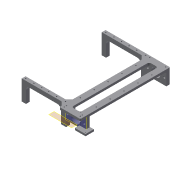
# Autodesk Inventor part: 02_Opentrons_Microscope_Base_v0
Saved by Autodesk Inventor 2019.4 (Build 234330000, 330)
## iProperties
Created: 2020-10-28
Part Number: 02_Opentrons_Microscope_Base_v0
Material: Generic
Document SubType Name: Modeling
Designer: diederichbenedict
Density: 1 g/cm^3
Appearance: Default
Author: diederichbenedict
Autodesk Inventor part; units mm, degrees
ref_plane "YZ Plane" through (0, 0, 0) normal (1, 0, 0) x (0, 1, 0)
ref_plane "XZ Plane" through (0, 0, 0) normal (0, 1, 0) x (-1, 0, 0)
ref_plane "XY Plane" through (0, 0, 0) normal (0, 0, 1) x (1, 0, 0)
ref_plane "Work Plane1" through (130.593, 54.6266, 280.0982) normal (0, 1, 0) x (1, 0, 0)
sketch "Sketch1" plane through (130.593, 54.6266, 280.0982) normal (0, 1, 0) x (1, 0, 0)
  line L0 (0, 36) -> (2, 38) projected
  line L1 (0, 27) -> (0, 36) projected
  line L2 (2, 25) -> (0, 27) projected
  line L3 (2, 25) -> (53, 25) projected
  line L4 (55, 27) -> (53, 25) projected
  line L5 (55, 27) -> (55, 36) projected
  line L6 (53, 38) -> (55, 36) projected
  line L7 (2, 38) -> (53, 38) projected
  circle A0 centre (6.5, 31.5) radius 2.5 construction
  circle A1 centre (48.5, 31.5) radius 2.5 construction
  line L8 (0, 224) -> (2, 226) projected
  line L9 (0, 215) -> (0, 224) projected
  line L10 (2, 213) -> (0, 215) projected
  line L11 (2, 213) -> (53, 213) projected
  line L12 (55, 215) -> (53, 213) projected
  line L13 (55, 215) -> (55, 224) projected
  line L14 (53, 226) -> (55, 224) projected
  line L15 (2, 226) -> (53, 226) projected
  circle A2 centre (6.5, 219.5) radius 2.5 construction
  circle A3 centre (48.5, 219.5) radius 2.5 construction
  line L16 (55, 25) -> (0, 25)
  line L17 (0, 25) -> (0, 261)
  line L18 (0, 261) -> (55, 261)
  line L19 (55, 261) -> (55, 25)
  line L20 (16, 261) -> (39, 261) projected
  circle A4 centre (48.5, 31.5) radius 1.45
  circle A5 centre (6.5, 31.5) radius 1.45
  circle A6 centre (48.5, 219.5) radius 1.45
  circle A7 centre (6.5, 219.5) radius 1.45
  point P0 (-130.593, 280.0982)
  dimension "d12" = 2.9
  dimension "d13" = 2.9
  dimension "d14" = 2.9
  dimension "d15" = 2.9
  constraints: 8 end point, 4 centre point, 3 coincident, 2 parallel, 2 point on line, 1 horizontal, 1 perpendicular
  measures "d12" diameter of A4
  measures "d13" diameter of A5
  measures "d14" diameter of A6
  measures "d15" diameter of A7
extrude "Extrusion1" add sketch "Sketch1" along normal blind 6
sketch "Sketch2" plane through (185.593, 54.6266, 19.0982) normal (0, 0, -1) x (-1, 0, 0)
  line L0 (46, 0) -> (46, 10) projected
  circle A0 centre (39, -26) radius 0.8 projected
  circle A1 centre (39, -3) radius 0.8 projected
  circle A2 centre (16, -26) radius 0.8 projected
  circle A3 centre (16, -3) radius 0.8 projected
  circle A4 centre (27.5, -14.5) radius 9.4 projected
  circle A5 centre (27.5, -14.5) radius 10.8 projected
  circle A6 centre (27.5, -14.5) radius 11.8
  circle A7 centre (5.5, -14.5) radius 3 projected
  circle A8 centre (49.5, -14.5) radius 3 projected
  circle A9 centre (5.5, -14.5) radius 3.1
  circle A10 centre (49.5, -14.5) radius 3.1
  line L1 (0, 0) -> (55, 0) projected
  line L2 (0, 0) -> (55, 0)
  line L3 (55, 0) -> (55, -32.5)
  line L4 (55, -32.5) -> (0, -32.5)
  line L5 (0, -32.5) -> (0, 0)
  point P0 (185.593, -54.6266)
  dimension "d2" = 1
  dimension "d3" = 6.2
  dimension "d4" = 6.2
  dimension "d5" = 18
  constraints: 8 end point, 3 centre point, 2 coincident, 2 parallel, 1 horizontal, 1 perpendicular
  measures "d2" radial gap between concentric circles of A5 A6
  measures "d3" diameter of A9
  measures "d4" diameter of A10
  measures "d5" distance from line of L4 A5.centre
extrude "Extrusion2" add sketch "Sketch2" against normal blind 10 contours L1 L3 L4 L5
ref_plane "Work Plane2" through (158.093, 40.1266, 239.5982) normal (0, 0, -1) x (1, 0, 0)
sketch "Sketch3" plane through (158.093, 40.1266, 239.5982) normal (0, 0, -1) x (1, 0, 0)
  circle A0 centre (-22, 0) radius 3 projected
  circle A1 centre (22, 0) radius 3 projected
  circle A2 centre (0, 0) radius 11.8 projected
  line L0 (27.5, -14.5) -> (27.5, -20.5) projected
  line L1 (-27.5, 18) -> (-27.5, -20.5) projected
  line L2 (27.5, -14.5) -> (-27.5, -14.5)
  line L3 (-27.5, -14.5) -> (-27.5, 15.5)
  line L4 (-27.5, 15.5) -> (27.5, 15.5)
  line L5 (27.5, 15.5) -> (27.5, -14.5)
  point P0 (-158.093, 40.1266)
  dimension "d51" = 30
  constraints: 8 end point, 2 parallel, 1 horizontal, 1 perpendicular, 1 point on line
  measures "d51" distance between parallel lines of L2 L4
extrude "Extrusion3" add sketch "Sketch3" along normal blind 10
fillet "Fillet1" radius 2 9 edges at (185.593, 41.3766, 19.0982) (158.093, 54.6266, 29.0982) (185.593, 39.6266, 229.5982) (185.593, 39.6266, 239.5982) (130.593, 39.6266, 229.5982) (130.593, 39.6266, 239.5982) (130.593, 57.6266, 255.0982) (185.593, 57.6266, 255.0982) (130.593, 41.3766, 19.0982)
sketch "Sketch4" plane through (130.593, 60.6266, 280.0982) normal (0, 1, 0) x (1, 0, 0)
  arc A0 (2, 261) -> (0, 259) centre (2, 259) ccw construction
  line L0 (0, 259) -> (0, 27) construction
  arc A1 (0, 27) -> (2, 25) centre (2, 27) ccw construction
  line L1 (2, 25) -> (53, 25) construction
  arc A2 (53, 25) -> (55, 27) centre (53, 27) ccw construction
  line L2 (55, 27) -> (55, 259) construction
  arc A3 (55, 259) -> (53, 261) centre (53, 259) ccw construction
  line L3 (53, 261) -> (2, 261) construction
  circle A4 centre (6.5, 219.5) radius 1.45 projected
  circle A5 centre (48.5, 219.5) radius 1.45 projected
  circle A6 centre (6.5, 31.5) radius 1.45 projected
  circle A7 centre (48.5, 31.5) radius 1.45 projected
  line L4 (16, 46) -> (16, 240)
  line L5 (21, 245) -> (34, 245)
  line L6 (39, 240) -> (39, 46)
  line L7 (34, 41) -> (21, 41)
  arc A8 (16, 46) -> (21, 41) centre (21, 46) ccw
  arc A9 (34, 41) -> (39, 46) centre (34, 46) ccw
  arc A10 (39, 240) -> (34, 245) centre (34, 240) ccw
  arc A11 (21, 245) -> (16, 240) centre (21, 240) ccw
  point P0 (-130.593, 280.0982)
  dimension "d16" = 16
  dimension "d17" = 5
  constraints: 8 end point, 8 point on circle, 8 tangent, 4 centre point, 3 equal radius, 3 other
  measures "d16" distance between parallel lines of L0 L4
  measures "d17" radius of A8
extrude "Extrusion4" cut sketch "Sketch4" against normal blind 25 contours L4 A11 L5 A10 L6 A9 L7 A8
sketch "Sketch5" plane through (130.593, 60.6266, 280.0982) normal (0, 1, 0) x (1, 0, 0)
  circle A0 centre (48.5, 219.5) radius 1.45 projected
  circle A1 centre (6.5, 219.5) radius 1.45 projected
  line L0 (0, 251) -> (55, 251) projected
  line L1 (0, 251) -> (55, 251) projected
  line L2 (0, 251) -> (55, 251) projected
  line L3 (16.8, 251) -> (15.2, 251) projected
  line L4 (16.8, 251) -> (15.2, 251) projected
  line L5 (39.8, 251) -> (38.2, 251) projected
  line L6 (39.8, 251) -> (38.2, 251) projected
  line L7 (52.6, 251) -> (46.4, 251) projected
  line L8 (8.6, 251) -> (2.4, 251) projected
  line L9 (39.3, 251) -> (15.7, 251) projected
  line L10 (53, 261) -> (2, 261) projected
  circle A2 centre (48.5, 256) radius 1.45
  circle A3 centre (6.5, 256) radius 1.45
  line L11 (55, 27) -> (55, 259) projected
  circle A4 centre (48.5, 219.5) radius 1.45
  circle A5 centre (6.5, 219.5) radius 1.45
  circle A6 centre (48.5, 183) radius 1.45
  circle A7 centre (6.5, 183) radius 1.45
  circle A8 centre (48.5, 146.5) radius 1.45
  circle A9 centre (6.5, 146.5) radius 1.45
  circle A10 centre (48.5, 110) radius 1.45
  circle A11 centre (6.5, 110) radius 1.45
  circle A12 centre (48.5, 73.5) radius 1.45
  circle A13 centre (6.5, 73.5) radius 1.45
  circle A14 centre (48.5, 37) radius 1.45
  circle A15 centre (6.5, 37) radius 1.45
  point P0 (-130.593, 280.0982)
  point P1 (53, 224.5)
  point P2 (55, 222.5)
  point P3 (2, 224.5)
  point P4 (53, 188)
  point P5 (55, 186)
  point P6 (2, 188)
  point P7 (53, 151.5)
  point P8 (55, 149.5)
  point P9 (2, 151.5)
  point P10 (53, 115)
  point P11 (55, 113)
  point P12 (2, 115)
  point P13 (53, 78.5)
  point P14 (55, 76.5)
  point P15 (2, 78.5)
  point P16 (53, 42)
  point P17 (55, 40)
  point P18 (2, 42)
  dimension "d20" = 2.9
  dimension "d21" = 2.9
  dimension "d22" = 5
  dimension "d23" = 5
  dimension "d24" = 36.5
  dimension "d27" = 36.5
  constraints: 14 centre point, 1 vertical, 42 other
  measures "d20" diameter of A2
  measures "d21" diameter of A3
  measures "d22" distance from line of A2.centre L10
  measures "d23" distance from line of L10 A3.centre
  measures "d24" distance of A0.centre A2.centre
  measures "d27" distance of L10.start point (53, 224.5)
extrude "Extrusion5" cut sketch "Sketch5" against normal through all contours A2 | A3 | A6 | A7 | A8 | A9 | A10 | A11 | A12 | A13 | A14 | A15
sketch "Sketch6" plane through (183.593, 22.1266, 19.0982) normal (0, 0, -1) x (-1, 0, 0)
  circle A0 centre (37, 6.5) radius 0.8 projected
  circle A1 centre (37, 29.5) radius 0.8 projected
  circle A2 centre (14, 6.5) radius 0.8 projected
  circle A3 centre (14, 29.5) radius 0.8 projected
  circle A4 centre (3.5, 18) radius 3.1 projected
  circle A5 centre (47.5, 18) radius 3.1 projected
  circle A6 centre (25.5, 18) radius 11.8 projected
  line L0 (51, 38.5) -> (51, 0) projected
  line L1 (0, 38.5) -> (51, 38.5) projected
  line L2 (0, 0) -> (0, 38.5) projected
  line L3 (0, 0) -> (51, 0) projected
  line L4 (167.6, -25.2) -> (167.6, -14.1084) construction
  line L5 (51, -25.2) -> (51, -14.1084) construction
  line L6 (167.6, -25.2) -> (51, -25.2) construction
  line L7 (167.6, 38.5) -> (51, 38.5)
  line L8 (51, 38.5) -> (51, -14.1084)
  line L9 (51, -14.1084) -> (167.6, -14.1084)
  line L10 (167.6, -14.1084) -> (167.6, 38.5)
  line L11 (156.5084, -14.1084) -> (156.5084, 17.4084)
  line L12 (146.5084, 27.4084) -> (74.0916, 27.4084)
  line L13 (64.0916, 17.4084) -> (64.0916, -14.1084)
  arc A7 (156.5084, 17.4084) -> (146.5084, 27.4084) centre (146.5084, 17.4084) ccw
  arc A8 (74.0916, 27.4084) -> (64.0916, 17.4084) centre (74.0916, 17.4084) ccw
  line L14 (51, -14.1084) -> (167.6, -14.1084) projected
  point P0 (183.593, -22.1266)
  point P1 (146.5084, -14.1084)
  point P2 (74.0916, -14.1084)
  point P3 (167.6, -14.1084)
  point P4 (51, -14.1084)
  dimension "d36" = 10
  constraints: 14 end point, 4 point on circle, 4 tangent, 3 perpendicular, 2 centre point, 2 parallel, 2 point on line, 1 equal radius, 1 horizontal, 1 vertical
  measures "d36" radius of A7
extrude "Extrusion6" add sketch "Sketch6" against normal up to surface (10 mm away) contours L7 L10 L9 L11 A7 L12 A8 L13 L8 L0
sketch "Sketch7" plane through (132.593, 54.6266, 239.5982) normal (0, 0, 1) x (1, 0, 0)
  circle A0 centre (14, -26) radius 0.8 construction
  circle A1 centre (14, -3) radius 0.8 construction
  circle A2 centre (37, -26) radius 0.8 construction
  circle A3 centre (37, -3) radius 0.8 construction
  circle A4 centre (47.5, -14.5) radius 3.1 construction
  circle A5 centre (3.5, -14.5) radius 3.1 projected
  circle A6 centre (25.5, -14.5) radius 11.8 projected
  line L0 (51, 6) -> (-116.6, 6) projected
  line L1 (51, -32.5) -> (51, 6) construction
  line L2 (51, -32.5) -> (0, -32.5) projected
  line L3 (0, -32.5) -> (0, -46.6084) projected
  line L4 (0, -46.6084) -> (-13.0916, -46.6084) projected
  line L5 (-13.0916, -46.6084) -> (-13.0916, -15.0916) projected
  arc A7 (-13.0916, -15.0916) -> (-23.0916, -5.0916) centre (-23.0916, -15.0916) ccw projected
  line L6 (-23.0916, -5.0916) -> (-95.5084, -5.0916) projected
  arc A8 (-95.5084, -5.0916) -> (-105.5084, -15.0916) centre (-95.5084, -15.0916) ccw projected
  line L7 (-105.5084, -15.0916) -> (-105.5084, -46.6084) projected
  line L8 (-105.5084, -46.6084) -> (-116.6, -46.6084) projected
  line L9 (-116.6, -46.6084) -> (-116.6, 6) projected
  line L10 (0, 0) -> (0, 6) projected
  line L11 (0, -32.5) -> (0, 6)
  point P0 (-132.593, -54.6266)
  constraints: 2 end point, 1 vertical
extrude "Extrusion7" add sketch "Sketch7" against normal blind 10 contours L10 L11 L3 L4 L5 A7 L6 A8 L7 L8 L9 L0
sketch "Sketch8" plane through (119.5013, 8.0182, 19.0982) normal (0, -1, 0) x (1, 0, 0)
  line L0 (-92.4167, 220.5) -> (-103.5084, 220.5) projected
  line L1 (-103.5084, 220.5) -> (-103.5084, 210.5) projected
  line L2 (-92.4167, 210.5) -> (-103.5084, 210.5) projected
  line L3 (-92.4167, 220.5) -> (-92.4167, 210.5) projected
  line L4 (13.0916, 210.5) -> (0, 210.5) projected
  line L5 (13.0916, 220.5) -> (0, 220.5) projected
  line L6 (0, 220.5) -> (0, 210.5) projected
  line L7 (13.0916, 220.5) -> (13.0916, 210.5) projected
  line L8 (-92.4167, 10) -> (-103.5084, 10) projected
  line L9 (-103.5084, 0) -> (-103.5084, 10) projected
  line L10 (-92.4167, 0) -> (-103.5084, 0) projected
  line L11 (-92.4167, 0) -> (-92.4167, 10) projected
  line L12 (13.0916, 10) -> (0, 10) projected
  line L13 (0, 0) -> (0, 10) projected
  line L14 (13.0916, 0) -> (0, 0) projected
  line L15 (13.0916, 0) -> (13.0916, 10) projected
  line L16 (-103.5084, 0) -> (13.0916, 0) projected
  line L17 (-0.1084, 10) -> (-99.5084, 10) projected
  circle A0 centre (-76.5084, 5) radius 1.45 projected
  circle A1 centre (-56.5084, 5) radius 1.45 projected
  circle A2 centre (-36.5084, 5) radius 1.45 projected
  circle A3 centre (-16.5084, 5) radius 1.45 projected
  line L18 (-10, 210.5) -> (-82.4167, 210.5) projected
  line L19 (-10, 220.5) -> (-82.4167, 220.5) projected
  point P0 (-119.5013, -19.0982)
  point P1 (-97.9625, 215.5)
  point P2 (6.5458, 215.5)
  point P3 (6.5458, 5)
  point P4 (-97.9625, 5)
  point P5 (-76.5084, 215.5)
  point P6 (-56.5084, 215.5)
  point P7 (-37.9584, 215.5)
  point P8 (-16.5084, 215.5)
hole "Hole1" at (21.5388, 8.0182, 234.5982) at (126.0472, 8.0182, 234.5982) at (126.0472, 8.0182, 24.0982) at (21.5388, 8.0182, 24.0982) at (42.993, 8.0182, 24.0982) at (62.993, 8.0182, 24.0982) at (82.993, 8.0182, 24.0982) at (102.993, 8.0182, 24.0982) at (42.993, 8.0182, 234.5982) at (62.993, 8.0182, 234.5982) at (81.543, 8.0182, 234.5982) at (102.993, 8.0182, 234.5982) direction (0, 1, 0) diameter 2.9 end through all counterbore diameter 7 counterbore depth 4
chamfer "Chamfer2" distance 10 angle 45 3 edges at (130.593, 57.6266, 229.5982) (130.593, 57.6266, 239.5982) (130.593, 56.6266, 29.0982)
sketch "Sketch9" plane through (185.593, 24.6266, 231.5982) normal (0, -1, 0) x (1, 0, 0)
  circle A0 centre (7, 16.9355) radius 1 construction
  circle A1 centre (-14.85, 7.2355) radius 1 construction
  line L0 (-17.85, 17.9355) -> (-17.85, 13.9936) construction
  line L1 (-17.85, 13.9936) -> (-25.5947, 13.9936) construction
  line L2 (-25.5947, 13.9936) -> (-25.5947, 12.9184) construction
  line L3 (-25.5947, 12.9184) -> (-17.85, 12.9184) construction
  line L4 (-17.85, 12.9184) -> (-17.85, 9.1835) construction
  line L5 (-17.85, 9.1835) -> (-25.5947, 9.1835) construction
  line L6 (-25.5947, 9.1835) -> (-25.5947, 8.5044) construction
  line L7 (-25.5947, 8.5044) -> (-17.85, 8.5044) construction
  line L8 (-17.85, 8.5044) -> (-17.85, 6.2355) construction
  arc A2 (-17.85, 6.2355) -> (-15.85, 4.2355) centre (-15.85, 6.2355) ccw construction
  line L9 (-15.85, 4.2355) -> (-10.3653, 4.2355) construction
  line L10 (-10.3653, 4.2355) -> (17.2162, -0.6279) construction
  line L11 (17.2162, -0.6279) -> (19.9478, -1.1095) projected
  line L12 (19.9478, -1.1095) -> (20, -0.8133) projected
  line L13 (20, -0.8133) -> (-8.6331, 4.2355) construction
  line L14 (-8.6331, 4.2355) -> (8, 4.2355) construction
  arc A3 (8, 4.2355) -> (10, 6.2355) centre (8, 6.2355) ccw construction
  line L15 (10, 6.2355) -> (10, 17.9355) construction
  arc A4 (10, 17.9355) -> (8, 19.9355) centre (8, 17.9355) ccw construction
  line L16 (8, 19.9355) -> (2.0209, 19.9355) construction
  line L17 (2.0209, 23.9533) -> (2.0209, 19.9355) construction
  line L18 (-6.5807, 23.9533) -> (2.0209, 23.9533) construction
  line L19 (-6.5807, 23.9533) -> (-6.5807, 22.9347) construction
  line L20 (-6.5807, 22.9347) -> (0.8325, 22.9347) construction
  line L21 (0.8325, 19.9355) -> (0.8325, 22.9347) construction
  line L22 (0.8325, 19.9355) -> (-15.85, 19.9355) construction
  arc A5 (-15.85, 19.9355) -> (-17.85, 17.9355) centre (-15.85, 17.9355) ccw construction
  line L23 (-2, -2) -> (-53, -2) projected
  line L24 (-16.5917, -2) -> (-38.4083, -2) projected
  line L25 (-17.85, -2) -> (10, -2)
  line L26 (10, -2) -> (10, 19.9355)
  line L27 (10, 19.9355) -> (-17.85, 19.9355)
  line L28 (-17.85, 19.9355) -> (-17.85, -2)
  circle A6 centre (-14.85, 7.2355) radius 1
  circle A7 centre (7, 16.9355) radius 1
  point P0 (-185.593, -231.5982)
  constraints: 8 end point, 2 centre point, 2 coincident, 2 parallel, 1 concentric, 1 horizontal, 1 perpendicular, 1 point on line
extrude "Extrusion8" add sketch "Sketch9" against normal blind 5
sketch "Sketch10" plane through (132.593, 24.6266, 229.5982) normal (0, -1, 0) x (1, 0, 0)
  circle A0 centre (38.15, 9.2355) radius 1 projected
  point P0 (-132.593, -229.5982)
extrude "Extrusion9" cut sketch "Sketch10" against normal through all
body "Solid1"
